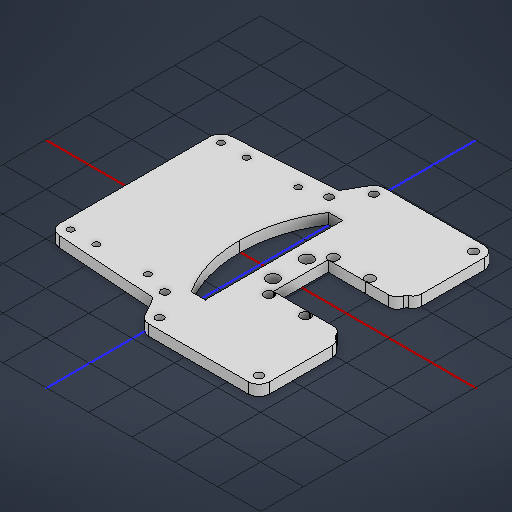
# Autodesk Inventor part: 000.010.005 - Резьбовая пластина
Saved by Autodesk Inventor 2025 (Build 290162000, 162)
## iProperties
Created: 2024-08-31
Part Number: 000.010.005 - Резьбовая пластина
Material: Типовые
Document SubType Name: Modeling
Designer: IvanPetrov
Density: 1 g/cm^3
Appearance: По умолчанию
Author: IvanPetrov
Autodesk Inventor part; units mm, degrees
ref_plane "YZ Plane" through (0, 0, 0) normal (1, 0, 0) x (0, 1, 0)
ref_plane "XZ Plane" through (0, 0, 0) normal (0, 1, 0) x (-1, 0, 0)
ref_plane "XY Plane" through (0, 0, 0) normal (0, 0, 1) x (1, 0, 0)
sketch "Эскиз1" plane through (0, 0, 0) normal (0, 1, 0) x (-1, 0, 0)
  circle A0 centre (53.024798, -34.512333) radius 1.5
  circle A1 centre (53.024798, 35.487667) radius 1.5
  circle A2 centre (41.024798, 35.487667) radius 1.5
  circle A3 centre (41.024798, -34.512333) radius 1.5
  circle A4 centre (17.024798, -34.512333) radius 1.5
  circle A5 centre (17.024798, 35.487667) radius 1.5
  circle A6 centre (5.8701, 38.795015) radius 1.85
  circle A7 centre (5.8701, -37.819681) radius 1.85
  circle A8 centre (-3.331957, -49.388251) radius 1.85
  circle A9 centre (-3.331957, 50.363585) radius 1.85
  circle A10 centre (-49.725202, 50.487667) radius 2
  circle A11 centre (-49.725202, -49.512333) radius 2
  circle A12 centre (53.024798, -34.512333) radius 5
  circle A13 centre (53.024798, 35.487667) radius 5
  circle A14 centre (5.8701, 38.795015) radius 5
  circle A15 centre (-49.725202, 50.487667) radius 5
  circle A16 centre (-3.331957, 50.363585) radius 5
  circle A17 centre (-49.725202, -49.512333) radius 5
  circle A18 centre (-3.331957, -49.388251) radius 5
  circle A19 centre (5.8701, -37.819681) radius 5
  line L0 (58.024798, -34.512333) -> (58.024798, 35.487667)
  line L1 (53.37463, 40.475414) -> (6.219932, 43.782761)
  line L2 (6.219932, 43.782761) -> (1.002517, 52.856041)
  line L3 (-3.318584, 55.363567) -> (-49.711829, 55.487649)
  line L4 (-54.725202, 50.487667) -> (-54.725202, -49.512333)
  line L5 (-50.00601, -54.504441) -> (-3.319511, -54.388236)
  line L6 (1.002517, -51.880707) -> (6.219932, -42.807427)
  line L7 (6.219932, -42.807427) -> (53.37463, -39.50008)
  arc A20 (9.274798, 0.487667) -> (-0.157574, 32.487667) centre (-49.725202, 0.486881) ccw
  arc A21 (-0.157574, -31.512333) -> (9.274798, 0.487667) centre (-49.725202, 0.488453) ccw
  line L8 (-6.725202, 32.487667) -> (-0.157574, 32.487667)
  line L9 (-6.725202, -31.512333) -> (-6.725202, 32.487667)
  line L10 (-0.157574, -31.512333) -> (-6.725202, -31.512333)
  circle A22 centre (-53.425202, 15.487667) radius 1.35
  circle A23 centre (-53.425202, 15.487667) radius 2.257107
  line L11 (-19.175202, 13.23056) -> (-63.375202, 13.23056)
  circle A24 centre (-36.425202, 15.487667) radius 1.35
  circle A25 centre (-36.425202, 15.487667) radius 2.26595
  circle A26 centre (-19.425202, 15.487667) radius 1.35
  circle A27 centre (-19.425202, 15.487667) radius 2.26595
  circle A28 centre (-13.925202, -7.587847) radius 1.35
  circle A29 centre (-13.925202, -7.587847) radius 2.853888
  circle A30 centre (-13.925202, 8.185931) radius 1.35
  circle A31 centre (-13.925202, 8.185931) radius 2.853888
  circle A32 centre (-19.425202, -14.512333) radius 1.35
  circle A33 centre (-19.425202, -14.512333) radius 2.257107
  line L12 (-63.375202, -12.255226) -> (-19.175202, -12.255226)
  circle A34 centre (-36.425202, -14.512333) radius 1.35
  circle A35 centre (-36.425202, -14.512333) radius 2.257107
  circle A36 centre (-53.425202, -14.512333) radius 1.35
  circle A37 centre (-53.425202, -14.512333) radius 2.257107
  line L13 (-19.175202, 13.23056) -> (-19.175202, -12.255226)
  point P0 (0, 0)
  point P1 (16.774798, 0.487667)
  point P2 (-54.725202, 17.332804)
  point P3 (-53.425202, 13.23056)
  point P4 (-36.625202, 13.23056)
  point P5 (-36.225202, 13.23056)
  point P6 (-19.625202, 13.23056)
  point P7 (-19.225202, 13.23056)
  point P8 (-19.425202, -12.255226)
  point P9 (-36.425202, -12.255226)
  point P10 (-53.425202, -12.255226)
  point P11 (-54.725202, -16.35747)
  dimension "d2" = 10
  dimension "d0" = 10
  dimension "d1" = 10
  dimension "d3" = 10
  dimension "d4" = 10
  dimension "d5" = 10
  dimension "d6" = 10
  dimension "d7" = 10
  constraints: 37 centre point, 28 end point, 18 point on circle, 16 coincident, 10 tangent, 1 vertical alignment, 4 other
  measures "d0" diameter of A12
  measures "d1" diameter of A13
  measures "d3" diameter of A15
  measures "d4" diameter of A16
  measures "d5" diameter of A17
  measures "d6" diameter of A18
  measures "d7" diameter of A19
sketch "Эскиз1 outline for Выдавливание1" plane through (0, 0, 0) normal (0, 1, 0) x (-1, 0, 0)
  arc A0 (53.37463, -39.50008) -> (58.024798, -34.512333) centre (53.024798, -34.512333) ccw
  line L0 (6.219932, -42.807427) -> (53.37463, -39.50008)
  line L1 (1.002517, -51.880707) -> (6.219932, -42.807427)
  arc A1 (-3.319511, -54.388236) -> (1.002517, -51.880707) centre (-3.331957, -49.388251) ccw
  line L2 (-50.00601, -54.504441) -> (-3.319511, -54.388236)
  arc A2 (-54.725202, -49.512333) -> (-50.00601, -54.504441) centre (-49.725202, -49.512333) ccw
  line L3 (-54.725202, -16.35747) -> (-54.725202, -49.512333)
  arc A3 (-53.425202, -12.255226) -> (-54.725202, -16.35747) centre (-53.425202, -14.512333) cw
  line L4 (-36.425202, -12.255226) -> (-53.425202, -12.255226)
  line L5 (-19.425202, -12.255226) -> (-36.425202, -12.255226)
  line L6 (-19.175202, -12.255226) -> (-19.425202, -12.255226)
  line L7 (-19.175202, 13.23056) -> (-19.175202, -12.255226)
  line L8 (-19.225202, 13.23056) -> (-19.175202, 13.23056)
  arc A4 (-19.625202, 13.23056) -> (-19.225202, 13.23056) centre (-19.425202, 15.487667) cw
  line L9 (-36.225202, 13.23056) -> (-19.625202, 13.23056)
  arc A5 (-36.625202, 13.23056) -> (-36.225202, 13.23056) centre (-36.425202, 15.487667) cw
  line L10 (-53.425202, 13.23056) -> (-36.625202, 13.23056)
  arc A6 (-54.725202, 17.332804) -> (-53.425202, 13.23056) centre (-53.425202, 15.487667) cw
  line L11 (-54.725202, 50.487667) -> (-54.725202, 17.332804)
  arc A7 (-49.711829, 55.487649) -> (-54.725202, 50.487667) centre (-49.725202, 50.487667) ccw
  line L12 (-3.318584, 55.363567) -> (-49.711829, 55.487649)
  arc A8 (1.002517, 52.856041) -> (-3.318584, 55.363567) centre (-3.331957, 50.363585) ccw
  line L13 (6.219932, 43.782761) -> (1.002517, 52.856041)
  line L14 (53.37463, 40.475414) -> (6.219932, 43.782761)
  arc A9 (58.024798, 35.487667) -> (53.37463, 40.475414) centre (53.024798, 35.487667) ccw
  line L15 (58.024798, -34.512333) -> (58.024798, 35.487667)
  circle A10 centre (-49.725202, -49.512333) radius 2
  circle A11 centre (-3.331957, -49.388251) radius 1.85
  arc A12 (-36.425202, -12.255226) -> (-34.168095, -14.512333) centre (-36.425202, -14.512333) ccw
  arc A13 (-34.168095, -14.512333) -> (-36.425202, -12.255226) centre (-36.425202, -14.512333) ccw
  arc A14 (-19.425202, -12.255226) -> (-17.168095, -14.512333) centre (-19.425202, -14.512333) ccw
  arc A15 (-17.168095, -14.512333) -> (-19.425202, -12.255226) centre (-19.425202, -14.512333) ccw
  circle A16 centre (-13.925202, -7.587847) radius 2.853888
  circle A17 centre (5.8701, -37.819681) radius 1.85
  circle A18 centre (17.024798, -34.512333) radius 1.5
  circle A19 centre (41.024798, -34.512333) radius 1.5
  circle A20 centre (53.024798, -34.512333) radius 1.5
  circle A21 centre (-13.925202, 8.185931) radius 2.853888
  line L16 (-0.157574, -31.512333) -> (-6.725202, -31.512333)
  arc A22 (9.274798, 0.487667) -> (-0.157574, -31.512333) centre (-49.725202, 0.488453) cw
  arc A23 (-0.157574, 32.487667) -> (9.274798, 0.487667) centre (-49.725202, 0.486881) cw
  line L17 (-6.725202, 32.487667) -> (-0.157574, 32.487667)
  line L18 (-6.725202, -31.512333) -> (-6.725202, 32.487667)
  circle A24 centre (-49.725202, 50.487667) radius 2
  circle A25 centre (-3.331957, 50.363585) radius 1.85
  circle A26 centre (5.8701, 38.795015) radius 1.85
  circle A27 centre (17.024798, 35.487667) radius 1.5
  circle A28 centre (41.024798, 35.487667) radius 1.5
  circle A29 centre (53.024798, 35.487667) radius 1.5
extrude "Выдавливание1" add sketch "Эскиз1 outline for Выдавливание1" along normal blind 5
fillet "Сопряжение1" radius 4 4 edges at (53.4252, 2.5, 13.2306) (54.7252, 2.5, 17.3328) (53.4252, 2.5, -12.2552) (54.7252, 2.5, -16.3575)
